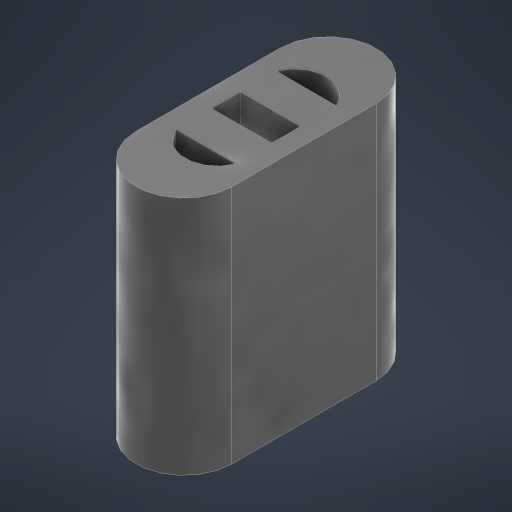
# Autodesk Inventor part: Pressure sensor connector
Saved by Autodesk Inventor 2023 (Build 270158000, 158)
## iProperties
Created: 2022-08-25
Part Number: Pressure sensor connector
Material: PET Plastic
Document SubType Name: Modeling
Designer: Mike
Density: 1.541 g/cm^3
Appearance: Fine Textured - Black
Author: Mike
Autodesk Inventor part; units mm, degrees
ref_plane "YZ Plane" through (0, 0, 0) normal (1, 0, 0) x (0, 1, 0)
ref_plane "XZ Plane" through (0, 0, 0) normal (0, 1, 0) x (-1, 0, 0)
ref_plane "XY Plane" through (0, 0, 0) normal (0, 0, 1) x (1, 0, 0)
sketch "Sketch1" plane through (0, 0, 0) normal (0, 1, 0) x (-1, 0, 0)
  line L0 (0, 5) -> (0, 5)
  line L1 (-2, 3) -> (-2, -3)
  line L2 (0, -5) -> (0, -5)
  line L3 (2, -3) -> (2, 3)
  line L4 (2, 5) -> (-2, -5) construction
  line L5 (-2, 5) -> (2, -5) construction
  arc A0 (2, 3) -> (0, 5) centre (0, 3) ccw
  arc A1 (0, -5) -> (2, -3) centre (0, -3) ccw
  arc A2 (-2, -3) -> (0, -5) centre (0, -3) ccw
  arc A3 (0, 5) -> (-2, 3) centre (0, 3) ccw
  line L6 (1.25, 0.6) -> (-1.25, 0.6)
  line L7 (-1.25, 0.6) -> (-1.25, -0.6)
  line L8 (-1.25, -0.6) -> (1.25, -0.6)
  line L9 (1.25, -0.6) -> (1.25, 0.6)
  line L10 (1.25, 0.6) -> (-1.25, -0.6) construction
  line L11 (-1.25, 0.6) -> (1.25, -0.6) construction
  arc A4 (-1.25, -2.1) -> (1.25, -2.1) centre (0, -1.6) ccw
  line L12 (-1.25, -2.1) -> (1.25, -2.1)
  line L13 (2, 0) -> (-2.9121, 0) construction
  arc A5 (1.25, 2.1) -> (-1.25, 2.1) centre (0, 1.6) ccw
  line L14 (-1.25, 2.1) -> (1.25, 2.1)
  point P0 (0, 0)
  dimension "d0" = 10
  dimension "d1" = 4
  dimension "d2" = 2
  dimension "d3" = 1.2
  dimension "d4" = 2.5
  dimension "d5" = 1.5
  dimension "d6" = 1.5
  dimension "d7" = 1
  dimension "d8" = 1.3463
  dimension "d9" = 0.75
  constraints: 30 end point, 12 point on circle, 8 point on line, 8 tangent, 6 centre point, 5 midpoint, 4 parallel, 3 equal radius, 3 horizontal, 3 symmetric about line, 2 perpendicular, 1 other
  measures "d0" distance of L5.start L4.end
  measures "d1" distance of L4.end L5.end
  measures "d2" radius of A0
  measures "d3" distance of L6.end L7.end
  measures "d4" distance of L7.end L8.end
  measures "d5" distance of L12.end L8.end
  measures "d6" distance of L12.start L7.end
  measures "d7" vertical distance of L7.end A4.centre
  measures "d8" radius of A4
  measures "d9" distance from line of L12.end L3
extrude "Extrusion1" add sketch "Sketch1" along normal blind 10
body "Solid1"
